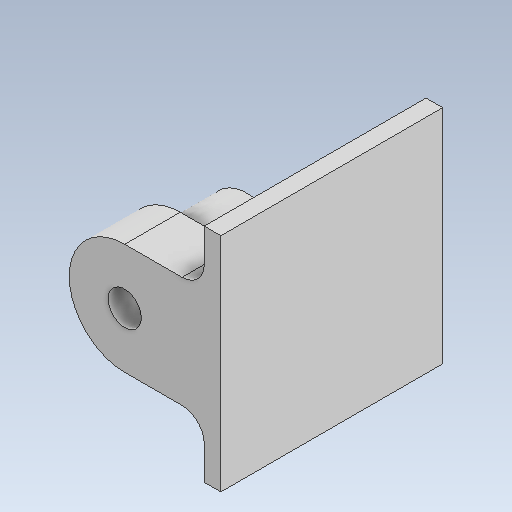
# Autodesk Inventor part: center_holder_boat
Saved by Autodesk Inventor 2020 (Build 240168000, 168)
## iProperties
Created: 2019-05-02
Part Number: center_holder_boat
Material: Generic
Document SubType Name: Modeling
Designer: erwin
Density: 1 g/cm^3
Appearance: Default
Author: erwin
Autodesk Inventor part; units mm, degrees
ref_plane "YZ Plane" through (0, 0, 0) normal (1, 0, 0) x (0, 1, 0)
ref_plane "XZ Plane" through (0, 0, 0) normal (0, 1, 0) x (-1, 0, 0)
ref_plane "XY Plane" through (0, 0, 0) normal (0, 0, 1) x (1, 0, 0)
sketch "Sketch1" plane through (0, 0, 0) normal (0, 0, 1) x (1, 0, 0)
  circle A0 centre (-2.2725, 0) radius 4 projected
  circle A1 centre (-2.2725, 0) radius 3.5
  point P0 (0, 0)
  dimension "d0" = 0.5
  constraints: 1 centre point
  measures "d0" radial gap between concentric circles of A0 A1
extrude "Extrusion1" add sketch "Sketch1" against normal blind 6 contours A1
sketch "Sketch2" plane through (-2.2725, 0, 0) normal (0, 0, 1) x (1, 0, 0)
  circle A0 centre (0, 0) radius 3.5 projected
  arc A1 (0, 5) -> (0, -5) centre (0, 0) ccw
  line L0 (0, 5) -> (7.1657, 5)
  line L1 (0, -5) -> (7.1657, -5)
  line L2 (8.6657, 10) -> (7.1657, 10)
  line L3 (7.1657, -10) -> (8.6657, -10)
  line L4 (8.6657, -10) -> (8.6657, 10)
  line L5 (7.1657, 10) -> (7.1657, 5)
  line L6 (7.1657, -5) -> (7.1657, -10)
  point P0 (2.2725, 0)
  dimension "d3" = 10
  dimension "d5" = 20
  dimension "d6" = 5
  dimension "d7" = 5
  dimension "d8" = 1.5
  dimension "d11" = 1.5
  constraints: 14 end point, 3 horizontal, 3 parallel, 2 perpendicular, 2 point on circle, 2 tangent, 1 centre point, 1 coincident
  measures "d3" diameter of A1
  measures "d5" distance of L3.end L2.start
  measures "d6" distance of L1.end L3.start
  measures "d7" distance of L2.end L0.end
  measures "d8" distance of L3.start L3.end
  measures "d11" distance of L2.start L2.end
extrude "Extrusion2" add sketch "Sketch2" along normal blind 5 contours A0 | L0 L5 L2 L4 L3 L6 L1 A1
sketch "Sketch3" plane through (-2.2725, 0, 0) normal (0, 0, -1) x (-1, 0, 0)
  arc A0 (0, -5) -> (0, 5) centre (0, 0) ccw projected
  line L0 (-7.1657, 5) -> (0, 5) projected
  line L1 (-7.1657, 10) -> (-7.1657, 5) projected
  line L2 (-8.6657, 10) -> (-7.1657, 10) projected
  line L3 (-8.6657, -10) -> (-8.6657, 10) projected
  line L4 (-7.1657, -10) -> (-8.6657, -10) projected
  line L5 (-7.1657, -5) -> (-7.1657, -10) projected
  line L6 (0, -5) -> (-7.1657, -5) projected
  circle A1 centre (0, 0) radius 3.5 projected
  line L7 (-7.1657, -5) -> (-7.1657, -10) projected
  line L8 (-7.1657, -5) -> (-7.1657, 5)
  point P0 (-2.2725, 0)
  constraints: 2 end point, 1 vertical
extrude "Extrusion3" add sketch "Sketch3" along normal blind 15 contours L5 L4 L3 L2 L1 L8
fillet "Fillet1" radius 2 2 edges at (4.8932, 5, 2.5) (4.8932, -5, 2.5)
sketch "Sketch4" plane through (-2.2725, 0, -6) normal (0, 0, -1) x (-1, 0, 0)
  circle A0 centre (0, 0) radius 3.5 projected
  point P0 (-2.2725, 0)
  constraints: 1 coincident
hole "Hole1" at (-2.2725, 0, -6) direction (0, 0, 1) diameter 3 end through all
equation "\"d7\" = d6"
equation "\"d11\" = d8"
body "Solid1"
